SteperMototrDriver v4 (Autodesk Fusion 360 design; units mm, degrees)
Autodesk Fusion 360 part; units mm, degrees
sketch "Sketch1" plane through (0, 0, 0) normal (0, 0, 1) x (1, 0, 0)
  line L0 (0, 0) -> (0, 12)
  line L1 (0, 12) -> (73, 12)
  line L2 (73, 12) -> (73, 34)
  line L3 (73, 34) -> (76, 34)
  line L4 (76, 34) -> (76, 0)
  line L5 (1, 0) -> (1, 9.5)
  line L6 (4, 9.5) -> (4, 0)
  line L7 (5, 9.5) -> (5, 0)
  line L8 (7.7368, 9.5) -> (7.7368, 0)
  line L9 (8.7368, 9.5) -> (8.7368, 0)
  line L10 (11.4737, 9.5) -> (11.4737, 0)
  line L11 (12.4737, 9.5) -> (12.4737, 0)
  line L12 (15.2105, 9.5) -> (15.2105, 0)
  line L13 (16.2105, 9.5) -> (16.2105, 0)
  line L14 (18.9474, 9.5) -> (18.9474, 0)
  line L15 (19.9474, 9.5) -> (19.9474, 0)
  line L16 (22.6842, 9.5) -> (22.6842, 0)
  line L17 (23.6842, 9.5) -> (23.6842, 0)
  line L18 (26.4211, 9.5) -> (26.4211, 0)
  line L19 (27.4211, 9.5) -> (27.4211, 0)
  line L20 (30.1579, 9.5) -> (30.1579, 0)
  line L21 (31.1579, 9.5) -> (31.1579, 0)
  line L22 (33.8947, 9.5) -> (33.8947, 0)
  line L23 (34.8947, 9.5) -> (34.8947, 0)
  line L24 (37.6316, 9.5) -> (37.6316, 0)
  line L25 (38.6316, 9.5) -> (38.6316, 0)
  line L26 (41.3684, 9.5) -> (41.3684, 0)
  line L27 (42.3684, 9.5) -> (42.3684, 0)
  line L28 (45.1053, 9.5) -> (45.1053, 0)
  line L29 (46.1053, 9.5) -> (46.1053, 0)
  line L30 (48.8421, 9.5) -> (48.8421, 0)
  line L31 (49.8421, 9.5) -> (49.8421, 0)
  line L32 (52.5789, 9.5) -> (52.5789, 0)
  line L33 (53.5789, 9.5) -> (53.5789, 0)
  line L34 (56.3158, 9.5) -> (56.3158, 0)
  line L35 (57.3158, 9.5) -> (57.3158, 0)
  line L36 (60.0526, 9.5) -> (60.0526, 0)
  line L37 (61.0526, 9.5) -> (61.0526, 0)
  line L38 (63.7895, 9.5) -> (63.7895, 0)
  line L39 (64.7895, 9.5) -> (64.7895, 0)
  line L40 (67.5263, 9.5) -> (67.5263, 0)
  line L41 (68.5263, 9.5) -> (68.5263, 0)
  line L42 (71.2632, 9.5) -> (71.2632, 0)
  line L43 (72.2632, 9.5) -> (72.2632, 0)
  line L44 (75, 9.5) -> (75, 0)
  line L45 (76, 9.5) -> (76, 0)
  line L46 (1, 0) -> (0, 0)
  line L47 (5, 0) -> (4, 0)
  line L48 (8.7368, 0) -> (7.7368, 0)
  line L49 (12.4737, 0) -> (11.4737, 0)
  line L50 (16.2105, 0) -> (15.2105, 0)
  line L51 (19.9474, 0) -> (18.9474, 0)
  line L52 (23.6842, 0) -> (22.6842, 0)
  line L53 (27.4211, 0) -> (26.4211, 0)
  line L54 (31.1579, 0) -> (30.1579, 0)
  line L55 (34.8947, 0) -> (33.8947, 0)
  line L56 (38.6316, 0) -> (37.6316, 0)
  line L57 (42.3684, 0) -> (41.3684, 0)
  line L58 (46.1053, 0) -> (45.1053, 0)
  line L59 (49.8421, 0) -> (48.8421, 0)
  line L60 (53.5789, 0) -> (52.5789, 0)
  line L61 (57.3158, 0) -> (56.3158, 0)
  line L62 (61.0526, 0) -> (60.0526, 0)
  line L63 (64.7895, 0) -> (63.7895, 0)
  line L64 (68.5263, 0) -> (67.5263, 0)
  line L65 (76, 0) -> (75, 0)
  line L66 (72.2632, 0) -> (71.2632, 0)
  line L67 (0, 9.5) -> (4, 9.5)
  line L68 (5, 9.5) -> (7.7368, 9.5)
  line L69 (8.7368, 9.5) -> (11.4737, 9.5)
  line L70 (12.4737, 9.5) -> (15.2105, 9.5)
  line L71 (16.2105, 9.5) -> (18.9474, 9.5)
  line L72 (19.9474, 9.5) -> (22.6842, 9.5)
  line L73 (23.6842, 9.5) -> (26.4211, 9.5)
  line L74 (27.4211, 9.5) -> (30.1579, 9.5)
  line L75 (31.1579, 9.5) -> (33.8947, 9.5)
  line L76 (34.8947, 9.5) -> (37.6316, 9.5)
  line L77 (38.6316, 9.5) -> (41.3684, 9.5)
  line L78 (42.3684, 9.5) -> (45.1053, 9.5)
  line L79 (46.1053, 9.5) -> (48.8421, 9.5)
  line L80 (49.8421, 9.5) -> (52.5789, 9.5)
  line L81 (53.5789, 9.5) -> (56.3158, 9.5)
  line L82 (57.3158, 9.5) -> (60.0526, 9.5)
  line L83 (61.0526, 9.5) -> (63.7895, 9.5)
  line L84 (64.7895, 9.5) -> (67.5263, 9.5)
  line L85 (68.5263, 9.5) -> (71.2632, 9.5)
  line L86 (72.2632, 9.5) -> (75, 9.5)
  dimension "d3723_1" = 12
  dimension "d3724_1" = 73
  dimension "d3725_1" = 3
  dimension "d3726_1" = 34
  dimension "d3727_1" = 2.5
  dimension "d3728_1" = 1
  dimension "d3729_1" = 1
  dimension "d3730_1" = 3
  dimension "d3733_1" = 71
  dimension "d3734_1" = 0
  constraint coincident L0.start L46.end
  constraint vertical L0
  constraint perpendicular L0 L1
  constraint perpendicular L1 L2
  constraint perpendicular L2 L3
  constraint perpendicular L3 L4
  constraint perpendicular L0 L65
  constraint coincident L0 L67.start
  constraint perpendicular L4 L67
  constraint coincident L5.start L65
  constraint coincident L5.end L67
  constraint perpendicular L5 L67
  constraint perpendicular L6 L65
  constraint coincident L7.start L67
  constraint coincident L7.end L65
  constraint perpendicular L7 L65
  constraint collinear L46 L65
  constraint collinear L47 L65
  constraint collinear L48 L65
  constraint collinear L49 L65
  constraint collinear L50 L65
  constraint collinear L51 L65
  constraint collinear L52 L65
  constraint collinear L53 L65
  constraint collinear L54 L65
  constraint collinear L55 L65
  constraint collinear L56 L65
  constraint collinear L57 L65
  constraint collinear L58 L65
  constraint collinear L59 L65
  constraint collinear L60 L65
  constraint collinear L61 L65
  constraint collinear L62 L65
  constraint collinear L63 L65
  constraint collinear L64 L65
  constraint collinear L65 L66
  constraint collinear L67 L68
  constraint collinear L68 L69
  constraint collinear L69 L70
  constraint collinear L70 L71
  constraint collinear L71 L72
  constraint collinear L72 L73
  constraint collinear L73 L74
  constraint collinear L74 L75
  constraint collinear L75 L76
  constraint collinear L76 L77
  constraint collinear L77 L78
  constraint collinear L78 L79
  constraint collinear L79 L80
  constraint collinear L80 L81
  constraint collinear L81 L82
  constraint collinear L82 L83
  constraint collinear L83 L84
  constraint collinear L84 L85
  constraint collinear L85 L86
  measures "d3723_1" distance of L0.start L0.end
  measures "d3724_1" distance of L0.end L1.end
  measures "d3725_1" distance of L2.end L3.end
  measures "d3726_1" distance of L3.end L4.end
  measures "d3727_1" distance of L1 L67
  measures "d3728_1" distance of L6 L7
  measures "d3729_1" distance of L0 L5
  measures "d3730_1" distance of L5 L6
extrude "Extrude1" add sketch "Sketch1" along normal blind 118 makes body 1
sketch "Sketch2" plane through (0, 0, 118) normal (0, 0, 1) x (-1, 0, 0)
  line L0 (-72.2632, 0) -> (-72.2632, -9.5)
  line L1 (-72.2632, -9.5) -> (-75, -9.5)
  line L2 (-75, -9.5) -> (-75, 0)
  line L3 (-75, 0) -> (-76, 0)
  line L4 (-76, 0) -> (-76, -34)
  line L5 (-76, -34) -> (-73, -34)
  line L6 (-73, -34) -> (-73, -12)
  line L7 (-73, -12) -> (0, -12)
  line L8 (0, -12) -> (0, 0)
  line L9 (0, 0) -> (-1, 0)
  line L10 (-1, 0) -> (-1, -9.5)
  line L11 (-1, -9.5) -> (-4, -9.5)
  line L12 (-4, -9.5) -> (-4, 0)
  line L13 (-4, 0) -> (-5, 0)
  line L14 (-5, 0) -> (-5, -9.5)
  line L15 (-5, -9.5) -> (-7.7368, -9.5)
  line L16 (-7.7368, -9.5) -> (-7.7368, 0)
  line L17 (-7.7368, 0) -> (-8.7368, 0)
  line L18 (-8.7368, 0) -> (-8.7368, -9.5)
  line L19 (-8.7368, -9.5) -> (-11.4737, -9.5)
  line L20 (-11.4737, -9.5) -> (-11.4737, 0)
  line L21 (-11.4737, 0) -> (-12.4737, 0)
  line L22 (-12.4737, 0) -> (-12.4737, -9.5)
  line L23 (-12.4737, -9.5) -> (-15.2105, -9.5)
  line L24 (-15.2105, -9.5) -> (-15.2105, 0)
  line L25 (-15.2105, 0) -> (-16.2105, 0)
  line L26 (-16.2105, 0) -> (-16.2105, -9.5)
  line L27 (-16.2105, -9.5) -> (-18.9474, -9.5)
  line L28 (-18.9474, -9.5) -> (-18.9474, 0)
  line L29 (-18.9474, 0) -> (-19.9474, 0)
  line L30 (-19.9474, 0) -> (-19.9474, -9.5)
  line L31 (-19.9474, -9.5) -> (-22.6842, -9.5)
  line L32 (-22.6842, -9.5) -> (-22.6842, 0)
  line L33 (-22.6842, 0) -> (-23.6842, 0)
  line L34 (-23.6842, 0) -> (-23.6842, -9.5)
  line L35 (-23.6842, -9.5) -> (-26.4211, -9.5)
  line L36 (-26.4211, -9.5) -> (-26.4211, 0)
  line L37 (-26.4211, 0) -> (-27.4211, 0)
  line L38 (-27.4211, 0) -> (-27.4211, -9.5)
  line L39 (-27.4211, -9.5) -> (-30.1579, -9.5)
  line L40 (-30.1579, -9.5) -> (-30.1579, 0)
  line L41 (-30.1579, 0) -> (-31.1579, 0)
  line L42 (-31.1579, 0) -> (-31.1579, -9.5)
  line L43 (-31.1579, -9.5) -> (-33.8947, -9.5)
  line L44 (-33.8947, -9.5) -> (-33.8947, 0)
  line L45 (-33.8947, 0) -> (-34.8947, 0)
  line L46 (-34.8947, 0) -> (-34.8947, -9.5)
  line L47 (-34.8947, -9.5) -> (-37.6316, -9.5)
  line L48 (-37.6316, -9.5) -> (-37.6316, 0)
  line L49 (-37.6316, 0) -> (-38.6316, 0)
  line L50 (-38.6316, 0) -> (-38.6316, -9.5)
  line L51 (-38.6316, -9.5) -> (-41.3684, -9.5)
  line L52 (-41.3684, -9.5) -> (-41.3684, 0)
  line L53 (-41.3684, 0) -> (-42.3684, 0)
  line L54 (-42.3684, 0) -> (-42.3684, -9.5)
  line L55 (-42.3684, -9.5) -> (-45.1053, -9.5)
  line L56 (-45.1053, -9.5) -> (-45.1053, 0)
  line L57 (-45.1053, 0) -> (-46.1053, 0)
  line L58 (-46.1053, 0) -> (-46.1053, -9.5)
  line L59 (-46.1053, -9.5) -> (-48.8421, -9.5)
  line L60 (-48.8421, -9.5) -> (-48.8421, 0)
  line L61 (-48.8421, 0) -> (-49.8421, 0)
  line L62 (-49.8421, 0) -> (-49.8421, -9.5)
  line L63 (-49.8421, -9.5) -> (-52.5789, -9.5)
  line L64 (-52.5789, -9.5) -> (-52.5789, 0)
  line L65 (-52.5789, 0) -> (-53.5789, 0)
  line L66 (-53.5789, 0) -> (-53.5789, -9.5)
  line L67 (-53.5789, -9.5) -> (-56.3158, -9.5)
  line L68 (-56.3158, -9.5) -> (-56.3158, 0)
  line L69 (-56.3158, 0) -> (-57.3158, 0)
  line L70 (-57.3158, 0) -> (-57.3158, -9.5)
  line L71 (-57.3158, -9.5) -> (-60.0526, -9.5)
  line L72 (-60.0526, -9.5) -> (-60.0526, 0)
  line L73 (-60.0526, 0) -> (-61.0526, 0)
  line L74 (-61.0526, 0) -> (-61.0526, -9.5)
  line L75 (-61.0526, -9.5) -> (-63.7895, -9.5)
  line L76 (-63.7895, -9.5) -> (-63.7895, 0)
  line L77 (-63.7895, 0) -> (-64.7895, 0)
  line L78 (-64.7895, 0) -> (-64.7895, -9.5)
  line L79 (-64.7895, -9.5) -> (-67.5263, -9.5)
  line L80 (-67.5263, -9.5) -> (-67.5263, 0)
  line L81 (-67.5263, 0) -> (-68.5263, 0)
  line L82 (-68.5263, 0) -> (-68.5263, -9.5)
  line L83 (-68.5263, -9.5) -> (-71.2632, -9.5)
  line L84 (-71.2632, -9.5) -> (-71.2632, 0)
  line L85 (-71.2632, 0) -> (-72.2632, 0)
  line L86 (0, -12) -> (0, -34)
  line L87 (0, -34) -> (-73, -34)
  constraint coincident L7.end L8.start
  constraint perpendicular L5 L86
  constraint coincident L5.end L6.start
  constraint perpendicular L6 L87
extrude "Extrude2" add sketch "Sketch2" against normal blind 118 separate body contours L6 L7 L86 L87 makes body 2
extrude "Extrude3" cut 1 faces at (24.3333, 26.6667, 0) along direction (0, 0, 1) blind 6.5 on bodies 2 bodies 2
extrude "Extrude4" cut 1 faces at (24.3333, 26.6667, 118) along direction (0, 0, -1) blind 6.5 on bodies 2 bodies 2
chamfer "Chamfer1" distance 4 angle 45 3 edges at (36.5, 34, 6.5) (0, 34, 59) (36.5, 34, 111.5) on bodies 2
sketch "Sketch3" plane through (73, 0, 0) normal (-1, 0, 0) x (0, -1, 0)
  line L0 (-34, 0) -> (-12, 0)
  line L1 (-12, 0) -> (-12, 118)
  line L2 (-12, 118) -> (-34, 118)
  line L3 (-34, 118) -> (-34, 0)
  line L4 (-21.5, 0) -> (-21.5, 118)
  line L5 (-26, 0) -> (-26, 118)
  line L6 (-26, 0) -> (-21.5, 0)
  line L7 (-23.75, 0) -> (-23.75, 3)
  circle A0 centre (-23.75, 3) radius 2.25
  line L8 (-26, 118) -> (-21.5, 118)
  line L9 (-23.75, 118) -> (-23.75, 115)
  circle A1 centre (-23.75, 115) radius 2.25
  dimension "d3744_1" = 9.5
  dimension "d3745_1" = 8
  dimension "d3746_1" = 3
  dimension "d3747_1" = 3
  constraint coincident L0 L4.start
  constraint coincident L2 L4.end
  constraint coincident L0 L5.start
  constraint perpendicular L0 L5
  constraint perpendicular L4 L6
  constraint midpoint L6 L7.start
  constraint perpendicular L6 L7
  constraint coincident L7.end A0.centre
  constraint tangent L5 A0
  constraint midpoint L8 L9.start
  constraint perpendicular L2 L9
  constraint coincident L9.end A1.centre
  constraint tangent L5 A1
  measures "d3744_1" distance of L0.end L4.start
  measures "d3745_1" distance of L3 L5
  measures "d3746_1" distance of L7.start L7.end
  measures "d3747_1" distance of L9.start L9.end
extrude "Extrude5" cut sketch "Sketch3" against normal blind 3 contours L0 L5 L6 L7 A0 | L0 L4 L6 L7 A0 | A0 | L2 L5 L8 L9 A1 | A1 | L2 L4 L8 L9 A1 bodies 1
sketch "Sketch4" plane through (0, 0, 0) normal (-1, 0, 0) x (0, -1, 0)
  line L0 (-30, 111.5) -> (-30, 6.5)
  line L1 (-30, 6.5) -> (-12, 6.5)
  line L2 (-12, 6.5) -> (-12, 111.5)
  line L3 (-12, 111.5) -> (-30, 111.5)
  line L4 (-20, 6.5) -> (-20, 111.5) construction
  line L5 (-34, 107.5) -> (-34, 10.5) construction
  line L6 (-20, 15.5) -> (-34, 15.5)
  line L7 (-34, 15.5) -> (-34, 46.5)
  line L8 (-34, 46.5) -> (-20, 46.5)
  line L9 (-20, 46.5) -> (-20, 15.5)
  line L10 (-20, 67.5) -> (-34, 67.5)
  line L11 (-34, 67.5) -> (-34, 98.5)
  line L12 (-34, 98.5) -> (-20, 98.5)
  line L13 (-20, 98.5) -> (-20, 67.5)
  line L14 (-30, 66.5) -> (-20, 66.5)
  line L15 (-20, 47.5) -> (-30, 47.5)
  line L16 (-20, 47.5) -> (-20, 66.5)
  dimension "d1" = 14
  dimension "d2" = 31
  dimension "d3" = 31
  dimension "d4" = 13
  dimension "d5" = 9
  dimension "d9" = 1
  dimension "d10" = 1
  constraint coincident L1 L4.start
  constraint coincident L3 L4.end
  constraint perpendicular L3 L4
  constraint horizontal L6
  constraint vertical L7
  constraint horizontal L8
  constraint vertical L9
  constraint coincident L5 L7.end
  constraint coincident L4 L6.start
  constraint horizontal L10
  constraint vertical L11
  constraint horizontal L12
  constraint vertical L13
  constraint coincident L5 L11.end
  constraint coincident L4 L10.start
  constraint coincident L0 L14.start
  constraint coincident L4 L14.end
  constraint perpendicular L4 L14
  constraint coincident L4 L15.start
  constraint coincident L0 L15.end
  constraint perpendicular L0 L15
  measures "d1" distance of L4 L5
  measures "d2" distance of L10.end L11.end
  measures "d3" distance of L6.end L7.end
  measures "d4" distance of L3 L12
  measures "d5" distance of L1 L6
  measures "d9" distance of L10.start L14.end
  measures "d10" distance of L8.end L15.start
extrude "Extrude6" add sketch "Sketch4" along normal blind 10 separate body contours L0 L10 L11 L12 | L0 L10 L12 L13 | L0 L6 L8 L9 | L0 L6 L7 L8 makes body 3 at (0, 29.3333, 77.8333) makes body 4 at (0, 29.3333, 36.1667)
chamfer "Chamfer2" distance 3 angle 45 2 edges at (0, 34, 31) (0, 34, 83) on bodies 3 4
extrude "Extrude7" add sketch "Sketch4" along normal blind 1 separate body contours L0 L14 L15 L16 makes body 5
equation "d3744_1 = 21.5 mm - 12 mm"
